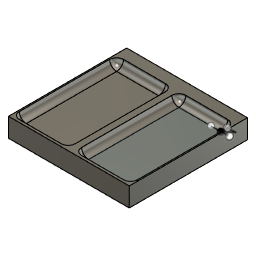
Suporte (Autodesk Fusion 360 design; units mm, degrees)
Autodesk Fusion 360 part; units mm, degrees
sketch "Esboço1" plane through (0, 0, 0) normal (0, 1, 0) x (1, 0, 0)
  line L0 (0, 0) -> (95, 0)
  line L1 (95, 0) -> (95, -93)
  line L2 (95, -93) -> (0, -93)
  line L3 (0, -93) -> (0, 0)
  dimension "d1" = 95
  dimension "d2" = 93
  constraint horizontal L0
  constraint vertical L1
  constraint horizontal L2
  constraint vertical L3
  constraint coincident L0.start L3.end
  measures "d1" distance of L0.start L0.end
  measures "d2" distance of L0.start L2.end
extrude "Extrusão1" add sketch "Esboço1" along normal blind 15
sketch "Esboço2" plane through (0, 15, 0) normal (0, 1, 0) x (-1, 0, 0)
  line L0 (0, 93) -> (-95, 93)
  line L1 (-95, 93) -> (-95, 0)
  line L2 (-95, 0) -> (0, 0)
  line L3 (0, 0) -> (0, 93)
  line L4 (-94, 91) -> (-50, 91)
  line L5 (-50, 91) -> (-50, 9)
  line L6 (-50, 9) -> (-94, 9)
  line L7 (-94, 9) -> (-94, 91)
  line L8 (-45, 91) -> (-1, 91)
  line L9 (-1, 91) -> (-1, 9)
  line L10 (-1, 9) -> (-45, 9)
  line L11 (-45, 9) -> (-45, 91)
  dimension "d10" = 44
  dimension "d11" = 82
  dimension "d12" = 44
  dimension "d13" = 82
  dimension "d14" = 1
  dimension "d15" = 1
  dimension "d16" = 5
  constraint horizontal L4
  constraint vertical L5
  constraint horizontal L6
  constraint vertical L7
  constraint horizontal L8
  constraint vertical L9
  constraint horizontal L10
  constraint vertical L11
  measures "d10" distance of L4.start L4.end
  measures "d11" distance of L4.start L6.end
  measures "d12" distance of L8.start L8.end
  measures "d13" distance of L8.start L10.end
  measures "d14" distance of L3 L9
  measures "d15" distance of L1 L7
  measures "d16" distance of L5 L11
extrude "Extrusão2" cut sketch "Esboço2" against normal blind 5.5 contours L4 L5 L6 L7 | L8 L9 L10 L11
fillet "Arredondamento2" radius 5.499 8 edges at (94, 9.5, 50) (72, 9.5, 91) (50, 9.5, 50) (72, 9.5, 9) (50, 12.25, 91) (94, 12.25, 91) (94, 12.25, 9) (50, 12.25, 9)
fillet "Arredondamento3" radius 5.4999 8 edges at (45, 9.5, 50) (23, 9.5, 9) (45, 12.25, 9) (45, 12.25, 91) (23, 9.5, 91) (1, 12.25, 91) (1, 9.5, 50) (1, 12.25, 9)
sketch "Esboço3" plane through (0, 9.5, 0) normal (0, 1, 0) x (-1, 0, 0)
  line L0 (-55.499, 14.499) -> (-55.499, 85.501)
  line L1 (-55.499, 85.501) -> (-88.501, 85.501)
  line L2 (-88.501, 85.501) -> (-88.501, 14.499)
  line L3 (-88.501, 14.499) -> (-55.499, 14.499)
  line L4 (-88.501, 14.499) -> (-93.501, 9.499)
  line L5 (-88.501, 14.499) -> (-80.8219, 14.499) construction
  line L6 (-93.501, 9.499) -> (-88.501, 9.499)
  line L7 (-88.501, 14.499) -> (-93.501, 14.499)
  line L8 (-93.501, 14.499) -> (-95, 14.499)
  line L9 (-89.7081, 13.999) -> (-93.8546, 9.8526)
  line L10 (-89.7081, 13.999) -> (-93.501, 13.999)
  line L11 (-93.501, 13.999) -> (-95, 13.999)
  line L12 (-93.501, 9.199) -> (-88.501, 9.199)
  line L13 (-93.8546, 9.8526) -> (-94.5081, 9.199)
  line L14 (-94.5081, 9.199) -> (-93.501, 9.199)
  dimension "d21" = 135
  dimension "d22" = 5
  dimension "d23" = -0.5
  dimension "d24" = 0.3
  constraint horizontal L5
  constraint coincident L2.end L3.start
  constraint perpendicular L2 L6
  constraint perpendicular L2 L7
  constraint parallel L7 L8
  constraint parallel L9 L13
  constraint parallel L12 L14
  measures "d21" angle of L4 L5
  measures "d22" distance of L2.end L6
